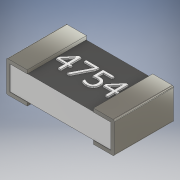
# Autodesk Inventor part: 21-1001
Saved by Autodesk Inventor 2018 (Build 220112000, 112)
## iProperties
Created: 2019-09-21
Part Number: 21-1001
Material: Copper
Document SubType Name: Modeling
Designer: Bradley
Density: 8.94 g/cm^3
Appearance: Smooth - White
Author: Bradley
Autodesk Inventor part; units mm, degrees
ref_plane "YZ Plane" through (0, 0, 0) normal (1, 0, 0) x (0, 1, 0)
ref_plane "XZ Plane" through (0, 0, 0) normal (0, 1, 0) x (-1, 0, 0)
ref_plane "XY Plane" through (0, 0, 0) normal (0, 0, 1) x (1, 0, 0)
sketch "Sketch1" plane through (0, 0, 0) normal (0, 1, 0) x (-1, 0, 0)
  line L0 (0.725, 0.175) -> (-0.725, 0.175)
  line L1 (-0.725, 0.175) -> (-0.725, -0.175)
  line L2 (-0.725, -0.175) -> (0.725, -0.175)
  line L3 (0.725, -0.175) -> (0.725, 0.175)
  line L4 (0.475, 0.175) -> (0.475, 0.225)
  line L5 (0.475, 0.225) -> (0.775, 0.225)
  line L6 (0.775, 0.225) -> (0.775, -0.225)
  line L7 (0.775, -0.225) -> (0.475, -0.225)
  line L8 (0.475, -0.225) -> (0.475, -0.175)
  line L9 (-0.475, 0.175) -> (-0.475, 0.225)
  line L10 (-0.475, 0.225) -> (-0.775, 0.225)
  line L11 (-0.775, 0.225) -> (-0.775, -0.225)
  line L12 (-0.775, -0.225) -> (-0.475, -0.225)
  line L13 (-0.475, -0.175) -> (-0.475, -0.225)
  line L14 (0.475, 0.175) -> (-0.475, 0.175)
  point P0 (0, 0)
  point P1 (0, 0.175)
  point P2 (0.725, 0)
  dimension "d0" = 1.55
  dimension "d1" = 0.05
  dimension "d2" = 0.05
  dimension "d3" = 0.45
  dimension "d4" = 0.3
  constraints: 30 end point, 12 point on line, 7 perpendicular, 3 collinear, 3 midpoint, 2 parallel, 1 horizontal, 1 horizontal alignment, 1 vertical, 1 vertical alignment
  measures "d0" distance between parallel lines of L11 L6
  measures "d1" distance of L7.end L8.end
  measures "d2" distance between parallel lines of L6 L3
  measures "d3" distance of L5.end L6.end
  measures "d4" distance of L6.end L7.end
extrude "Extrusion1" add sketch "Sketch1" along normal mid plane 0.85 contours L0 L4 L5 L6 L7 L8 L2 L3 | L0 L1 L2 L13 L12 L11 L10 L9
extrude "Extrusion2" add sketch "Sketch1" along normal mid plane 0.84 contours L3 L2 L1 L0
sketch "Sketch2" plane through (-0.475, -0.42, 0.175) normal (0, 0, 1) x (1, 0, 0)
  line L0 (0, 0) -> (0, 0.84) projected
  line L1 (0.95, 0) -> (0, 0) projected
  line L2 (0.95, 0) -> (0.95, 0.84) projected
  line L3 (0, 0.84) -> (0.95, 0.84) projected
  line L4 (0, 0.42) -> (0.95, 0.42) construction
  line L5 (0.2397, 0.3731) -> (0.2039, 0.3731)
  line L6 (0.2039, 0.3731) -> (0.2039, 0.27)
  line L7 (0.2039, 0.27) -> (0.1653, 0.27)
  line L8 (0.1653, 0.27) -> (0.1653, 0.3731)
  line L9 (0.1653, 0.3731) -> (0.0328, 0.3731)
  line L10 (0.0328, 0.3731) -> (0.0328, 0.4154)
  line L11 (0.0328, 0.4154) -> (0.167, 0.57)
  line L12 (0.167, 0.57) -> (0.2039, 0.57)
  line L13 (0.2039, 0.57) -> (0.2039, 0.4054)
  line L14 (0.2039, 0.4054) -> (0.2397, 0.4054)
  line L15 (0.2397, 0.4054) -> (0.2397, 0.3731)
  line L16 (0.1653, 0.4054) -> (0.1653, 0.5226)
  line L17 (0.1653, 0.5226) -> (0.0644, 0.4054)
  line L18 (0.0644, 0.4054) -> (0.1653, 0.4054)
  line L19 (0.4602, 0.525) -> (0.3303, 0.27)
  line L20 (0.3303, 0.27) -> (0.2876, 0.27)
  line L21 (0.2876, 0.27) -> (0.4247, 0.5347)
  line L22 (0.4247, 0.5347) -> (0.2698, 0.5347)
  line L23 (0.2698, 0.5347) -> (0.2698, 0.57)
  line L24 (0.2698, 0.57) -> (0.4602, 0.57)
  line L25 (0.4602, 0.57) -> (0.4602, 0.525)
  spline S0 degree 2 poles (0.6787, 0.3653) (0.6787, 0.3437) (0.6649, 0.3067) (0.6522, 0.2931) knots 0 0 0 1 2 2 2
  spline S1 degree 2 poles (0.6522, 0.2931) (0.6396, 0.2795) (0.6019, 0.2637) (0.5786, 0.2637) knots 0 0 0 1 2 2 2
  spline S2 degree 2 poles (0.5786, 0.2637) (0.5572, 0.2637) (0.5154, 0.2732) (0.5, 0.2807) knots 0 0 0 1 2 2 2
  line L26 (0.5, 0.2807) -> (0.5, 0.3232)
  line L27 (0.5, 0.3232) -> (0.503, 0.3232)
  spline S3 degree 2 poles (0.503, 0.3232) (0.5076, 0.3198) (0.5248, 0.3111) (0.5353, 0.3072) knots 0 0 0 1 2 2 2
  spline S4 degree 2 poles (0.5353, 0.3072) (0.5472, 0.3031) (0.5669, 0.2984) (0.5793, 0.2984) knots 0 0 0 1 2 2 2
  spline S5 degree 2 poles (0.5793, 0.2984) (0.5915, 0.2984) (0.6143, 0.3072) (0.6226, 0.3167) knots 0 0 0 1 2 2 2
  spline S6 degree 2 poles (0.6226, 0.3167) (0.6301, 0.3257) (0.6379, 0.3495) (0.6379, 0.3655) knots 0 0 0 1 2 2 2
  spline S7 degree 2 poles (0.6379, 0.3655) (0.6379, 0.3816) (0.6291, 0.402) (0.6209, 0.4088) knots 0 0 0 1 2 2 2
  spline S8 degree 2 poles (0.6209, 0.4088) (0.6124, 0.4164) (0.5871, 0.4227) (0.5718, 0.4227) knots 0 0 0 1 2 2 2
  spline S9 degree 2 poles (0.5718, 0.4227) (0.5552, 0.4227) (0.5224, 0.4176) (0.5124, 0.4154) knots 0 0 0 1 2 2 2
  line L28 (0.5124, 0.4154) -> (0.5124, 0.57)
  line L29 (0.5124, 0.57) -> (0.677, 0.57)
  line L30 (0.677, 0.57) -> (0.677, 0.5347)
  line L31 (0.677, 0.5347) -> (0.5511, 0.5347)
  line L32 (0.5511, 0.5347) -> (0.5511, 0.4548)
  spline S10 degree 2 poles (0.5511, 0.4548) (0.5584, 0.4557) (0.5725, 0.4565) (0.5783, 0.4565) knots 0 0 0 1 2 2 2
  spline S11 degree 2 poles (0.5783, 0.4565) (0.6014, 0.4565) (0.6333, 0.4489) (0.6479, 0.4377) knots 0 0 0 1 2 2 2
  spline S12 degree 2 poles (0.6479, 0.4377) (0.6627, 0.4266) (0.6787, 0.3925) (0.6787, 0.3653) knots 0 0 0 1 2 2 2
  line L33 (0.915, 0.3731) -> (0.8793, 0.3731)
  line L34 (0.8793, 0.3731) -> (0.8793, 0.27)
  line L35 (0.8793, 0.27) -> (0.8406, 0.27)
  line L36 (0.8406, 0.27) -> (0.8406, 0.3731)
  line L37 (0.8406, 0.3731) -> (0.7081, 0.3731)
  line L38 (0.7081, 0.3731) -> (0.7081, 0.4154)
  line L39 (0.7081, 0.4154) -> (0.8423, 0.57)
  line L40 (0.8423, 0.57) -> (0.8793, 0.57)
  line L41 (0.8793, 0.57) -> (0.8793, 0.4054)
  line L42 (0.8793, 0.4054) -> (0.915, 0.4054)
  line L43 (0.915, 0.4054) -> (0.915, 0.3731)
  line L44 (0.8406, 0.4054) -> (0.8406, 0.5226)
  line L45 (0.8406, 0.5226) -> (0.7397, 0.4054)
  line L46 (0.7397, 0.4054) -> (0.8406, 0.4054)
  point P0 (0.475, 0.42)
  constraints: 2 end point, 2 midpoint, 1 horizontal
extrude "Extrusion3" add sketch "Sketch2" along normal blind 0.02 contours L5 L6 L7 L8 L9 L10 L11 L12 L13 L14 L15 | L19 L20 L21 L22 L23 L24 L25 | S0 S1 S2 L26 L27 S3 S4 S5 S6 S7 S8 S9 L28 L29 L30 L31 L32 S10 S11 S12 | L33 L34 L35 L36 L37 L38 L39 L40 L41 L42 L43
fillet "Fillet1" radius 0.02 4 edges at (-0.775, 0, 0.225) (-0.775, 0, -0.225) (0.775, 0, 0.225) (0.775, 0, -0.225)
equation "\"d2\" = d1"
body "Solid1"
